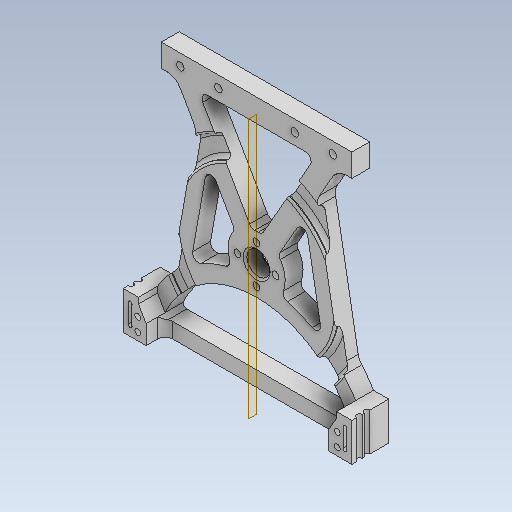
# Autodesk Inventor part: drv_stand_1
Saved by Autodesk Inventor 2020 (Build 240168000, 168)
## iProperties
Created: 2021-08-05
Part Number: drv_stand_1
Material: Generic
Document SubType Name: Modeling
Designer: Shuang Peng
Density: 1 g/cm^3
Appearance: Default
Author: Shuang Peng
Autodesk Inventor part; units mm, degrees
ref_plane "YZ Plane" through (0, 0, 0) normal (1, 0, 0) x (0, 1, 0)
ref_plane "XZ Plane" through (0, 0, 0) normal (0, 1, 0) x (-1, 0, 0)
ref_plane "XY Plane" through (0, 0, 0) normal (0, 0, 1) x (1, 0, 0)
sketch "Sketch1" plane through (0, 0, 0) normal (0, 0, 1) x (1, 0, 0)
  circle A0 centre (6, 23) radius 1.6 projected
  circle A1 centre (-6, 23) radius 1.6 projected
  arc A2 (-0.5, 30.4959) -> (0.5, 30.4959) centre (0, 0) ccw projected
  line L0 (0.5, 30.4959) -> (0.5, 11) projected
  arc A3 (-0.5, 11) -> (0.5, 11) centre (0, 11) ccw projected
  line L1 (-0.5, 11) -> (-0.5, 30.4959) projected
  circle A4 centre (-7, 0) radius 1.6 projected
  circle A5 centre (0, 7) radius 1.6 projected
  circle A6 centre (0, -7) radius 1.6 projected
  circle A7 centre (7, 0) radius 1.6 projected
  line L2 (-9.2147, 23.438) -> (-5.6564, 9.7982) projected
  arc A8 (-6.3264, 7.7445) -> (-5.6564, 9.7982) centre (-7.5917, 9.2933) ccw projected
  arc A9 (-6.3264, 7.7445) -> (-9.5652, 2.9167) centre (0, 0) ccw projected
  arc A10 (-11.4782, 1.5) -> (-9.5652, 2.9167) centre (-11.4782, 3.5) ccw projected
  line L3 (-11.4782, 1.5) -> (-25.2587, 1.5) projected
  arc A11 (-27.2397, 3.7745) -> (-25.2587, 1.5) centre (-25.2587, 3.5) ccw projected
  arc A12 (-12.0244, 24.7318) -> (-27.2397, 3.7745) centre (0, 0) ccw projected
  arc A13 (-9.2147, 23.438) -> (-12.0244, 24.7318) centre (-11.1499, 22.9332) ccw projected
  line L4 (-1.5, -11.4782) -> (-1.5, -25.2587) projected
  arc A14 (-3.7745, -27.2397) -> (-1.5, -25.2587) centre (-3.5, -25.2587) ccw projected
  arc A15 (-27.2397, -3.7745) -> (-3.7745, -27.2397) centre (0, 0) ccw projected
  arc A16 (-25.2587, -1.5) -> (-27.2397, -3.7745) centre (-25.2587, -3.5) ccw projected
  line L5 (-25.2587, -1.5) -> (-11.4782, -1.5) projected
  arc A17 (-9.5652, -2.9167) -> (-11.4782, -1.5) centre (-11.4782, -3.5) ccw projected
  arc A18 (-9.5652, -2.9167) -> (-2.9167, -9.5652) centre (0, 0) ccw projected
  arc A19 (-1.5, -11.4782) -> (-2.9167, -9.5652) centre (-3.5, -11.4782) ccw projected
  line L6 (5.6564, 9.7982) -> (9.2147, 23.438) projected
  arc A20 (12.0244, 24.7318) -> (9.2147, 23.438) centre (11.1499, 22.9332) ccw projected
  arc A21 (27.2397, 3.7745) -> (12.0244, 24.7318) centre (0, 0) ccw projected
  arc A22 (25.2587, 1.5) -> (27.2397, 3.7745) centre (25.2587, 3.5) ccw projected
  line L7 (25.2587, 1.5) -> (11.4782, 1.5) projected
  arc A23 (9.5652, 2.9167) -> (11.4782, 1.5) centre (11.4782, 3.5) ccw projected
  arc A24 (9.5652, 2.9167) -> (6.3264, 7.7445) centre (0, 0) ccw projected
  arc A25 (5.6564, 9.7982) -> (6.3264, 7.7445) centre (7.5917, 9.2933) ccw projected
  line L8 (1.5, -25.2587) -> (1.5, -11.4782) projected
  arc A26 (2.9167, -9.5652) -> (1.5, -11.4782) centre (3.5, -11.4782) ccw projected
  arc A27 (2.9167, -9.5652) -> (9.5652, -2.9167) centre (0, 0) ccw projected
  arc A28 (11.4782, -1.5) -> (9.5652, -2.9167) centre (11.4782, -3.5) ccw projected
  line L9 (11.4782, -1.5) -> (25.2587, -1.5) projected
  arc A29 (27.2397, -3.7745) -> (25.2587, -1.5) centre (25.2587, -3.5) ccw projected
  arc A30 (3.7745, -27.2397) -> (27.2397, -3.7745) centre (0, 0) ccw projected
  arc A31 (1.5, -25.2587) -> (3.7745, -27.2397) centre (3.5, -25.2587) ccw projected
  circle A32 centre (0, 0) radius 2 projected
  line L10 (0, 0) -> (-30, 0)
  line L11 (-30, 0) -> (-30, -20)
  line L12 (-30, -20) -> (-30, -28)
  line L13 (-30, -28) -> (-26, -28)
  line L14 (-26, -28) -> (-26, -18)
  line L15 (-26, -18) -> (-30, -18)
  line L16 (-30, -18) -> (-30, -28)
  dimension "d0" = 30
  dimension "d1" = 20
  dimension "d2" = 8
  dimension "d3" = 4
  dimension "d4" = 10
  constraints: 14 end point, 2 horizontal, 2 parallel, 2 vertical, 1 perpendicular
  measures "d0" distance of L10.start L10.end
  measures "d1" distance of L10.end L11.end
  measures "d2" distance of L11.end L12.end
  measures "d3" distance of L15.end L14.end
  measures "d4" distance of L14.end L13.end
ref_plane "Work Plane1" through (-30.5, -30.5, -4) normal (0, 0, -1) x (0, 1, 0)
extrude "Extrusion1" add sketch "Sketch1" against normal up to surface (4 mm away) contours L15 L14 L13 L12 L11
sketch "Sketch2" plane through (-26, -28, -4) normal (0, 0, -1) x (-1, 0, 0)
  line L0 (4, 0) -> (0, 0) projected
  line L1 (4, 10) -> (4, 0) projected
  line L2 (0, 10) -> (4, 10) projected
  line L3 (0, 0) -> (0, 10) projected
  line L4 (4, 0) -> (0, 0) projected
  line L5 (0, 0) -> (-2, 0)
  line L6 (-2, 0) -> (-2, 5)
  line L7 (-2, 5) -> (0, 8.4641)
  line L8 (0, 0) -> (0, 10) projected
  point P0 (-26, 28)
  point P1 (0, 8.4641)
  dimension "d7" = 2
  dimension "d8" = 5
  dimension "d9" = 30
  constraints: 6 end point, 1 horizontal, 1 parallel, 1 point on line
  measures "d7" distance of L0.end L5.end
  measures "d8" distance of L5.end L6.end
  measures "d9" angle of L3 L7
extrude "Extrusion2" add sketch "Sketch2" against normal up to surface (4 mm away) contours L5 L6 L7 L3
sketch "Sketch3" plane through (-26, -18, -4) normal (0, 0, -1) x (-1, 0, 0)
  line L0 (4, -10) -> (-2, -10) projected
  line L1 (4, 0) -> (4, -10) projected
  line L2 (0, 0) -> (4, 0) projected
  line L3 (0, -1.5359) -> (0, 0) projected
  line L4 (0, -1.5359) -> (-2, -5) projected
  line L5 (-2, -5) -> (-2, -10) projected
  line L6 (4, -10) -> (-2, -10) projected
  line L7 (-2, -10) -> (0.2, -10)
  line L8 (0.2, -10) -> (0.2, -8)
  line L9 (0.2, -8) -> (0.2, -4.5)
  circle A0 centre (0.2, -4.5) radius 0.75
  circle A1 centre (0.2, -8) radius 0.75
  point P0 (-26, 18)
  dimension "d12" = 2.2
  dimension "d13" = 2
  dimension "d14" = 3.5
  dimension "d15" = 1.5
  dimension "d16" = 1.5
  constraints: 6 end point, 2 centre point, 2 coincident, 2 point on line, 1 vertical
  measures "d12" distance of L0.end L7.end
  measures "d13" distance of L7.end L8.end
  measures "d14" distance of L8.end L9.end
  measures "d15" diameter of A0
  measures "d16" diameter of A1
extrude "Extrusion3" cut sketch "Sketch3" against normal blind 10 contours A1 L9 L8 | L8 L9 A1 | A0
ref_plane "Work Plane2" through (0, 30.996, -2) normal (-1, 0, 0) x (0, -1, 0)
mirror "Mirror1" about plane through (0, 30.996, -2) normal (-1, 0, 0) of "Extrusion1", "Extrusion2", "Extrusion3"
sketch "Sketch4" plane through (24, -28, -4) normal (0, 0, -1) x (-1, 0, 0)
  circle A0 centre (24, 28) radius 3.05
  circle A1 centre (24, 28) radius 7.5
  circle A2 centre (-2.2, 2) radius 0.75 projected
  circle A3 centre (-2.2, 5.5) radius 0.75 projected
  line L0 (-6, 0) -> (0, 0) projected
  line L1 (0, 5) -> (0, 0) projected
  line L2 (-2, 8.4641) -> (0, 5) projected
  line L3 (-2, 8.4641) -> (-2, 10) projected
  line L4 (-2, 10) -> (-6, 10) projected
  line L5 (-6, 10) -> (-6, 0) projected
  line L6 (54, 10) -> (54, 0) projected
  circle A4 centre (50.2, 2) radius 0.75 projected
  circle A5 centre (50.2, 5.5) radius 0.75 projected
  line L7 (54, 0) -> (48, 0) projected
  line L8 (54, 10) -> (54, 0) projected
  line L9 (50, 10) -> (54, 10) projected
  line L10 (50, 8.4641) -> (50, 10) projected
  line L11 (50, 8.4641) -> (48, 5) projected
  line L12 (48, 5) -> (48, 0) projected
  line L13 (0, 5) -> (0, 0) projected
  arc A6 (48, 5) -> (0, 5) centre (24, -5.8306) ccw
  line L14 (50, 10) -> (54, 10) projected
  line L15 (-2, 8.4641) -> (-2, 10) projected
  arc A7 (50, 10) -> (-2, 10) centre (24, -5.8306) ccw
  point P0 (30.3113, 23.9482)
  point P1 (17.6887, 23.9482)
  dimension "d19" = 6.1
  dimension "d20" = 15
  constraints: 4 centre point, 4 point on circle, 2 coincident, 1 concentric, 1 tangent
  measures "d19" diameter of A0
  measures "d20" diameter of A1
extrude "Extrusion4" add sketch "Sketch4" along normal blind 3
sketch "Sketch5" plane through (24, -28, -7) normal (0, 0, -1) x (-1, 0, 0)
  arc A0 (48, 5) -> (0, 5) centre (24, -5.8306) ccw projected
  line L0 (48, 5) -> (48, 0) projected
  line L1 (48, 0) -> (54, 0) projected
  line L2 (54, 0) -> (54, 10) projected
  line L3 (54, 10) -> (50, 10) projected
  arc A1 (50, 10) -> (30.3113, 23.9482) centre (24, -5.8306) ccw projected
  arc A2 (30.3113, 23.9482) -> (17.6887, 23.9482) centre (24, 28) ccw projected
  arc A3 (17.6887, 23.9482) -> (-2, 10) centre (24, -5.8306) ccw projected
  line L4 (-2, 10) -> (-6, 10) projected
  line L5 (-6, 10) -> (-6, 0) projected
  line L6 (-6, 0) -> (0, 0) projected
  line L7 (0, 0) -> (0, 5) projected
  circle A4 centre (24, 28) radius 3.05 projected
  circle A5 centre (50.2, 2) radius 0.75 projected
  circle A6 centre (50.2, 5.5) radius 0.75 projected
  circle A7 centre (-2.2, 5.5) radius 0.75 projected
  circle A8 centre (-2.2, 2) radius 0.75 projected
  circle A9 centre (24, 28) radius 5.55
  dimension "d23" = 2.5
  constraints: 1 centre point, 1 coincident
  measures "d23" radial gap between concentric circles of A4 A9
extrude "Extrusion5" add sketch "Sketch5" along normal blind 4 contours A9
sketch "Sketch6" plane through (24, -28, -7) normal (0, 0, -1) x (-1, 0, 0)
  circle A0 centre (24, 28) radius 5.55 projected
  arc A1 (48, 5) -> (0, 5) centre (24, -5.8306) ccw projected
  line L0 (48, 5) -> (48, 0) projected
  line L1 (48, 0) -> (54, 0) projected
  line L2 (54, 0) -> (54, 10) projected
  line L3 (54, 10) -> (50, 10) projected
  arc A2 (50, 10) -> (30.3113, 23.9482) centre (24, -5.8306) ccw projected
  arc A3 (30.3113, 23.9482) -> (17.6887, 23.9482) centre (24, 28) ccw projected
  arc A4 (17.6887, 23.9482) -> (-2, 10) centre (24, -5.8306) ccw projected
  line L4 (-2, 10) -> (-6, 10) projected
  line L5 (-6, 10) -> (-6, 0) projected
  line L6 (-6, 0) -> (0, 0) projected
  line L7 (0, 0) -> (0, 5) projected
  circle A5 centre (50.2, 2) radius 0.75 projected
  circle A6 centre (50.2, 5.5) radius 0.75 projected
  circle A7 centre (-2.2, 5.5) radius 0.75 projected
  circle A8 centre (-2.2, 2) radius 0.75 projected
  line L8 (-6, 0) -> (0, 0) projected
  line L9 (0, 0) -> (48, 0)
  line L10 (48, 0) -> (48, 4)
  line L11 (48, 4) -> (0, 4)
  line L12 (0, 4) -> (0, 0)
  point P0 (0, 4)
  dimension "d26" = 4
  constraints: 8 end point, 2 parallel, 1 horizontal, 1 perpendicular, 1 point on line
  measures "d26" distance between parallel lines of L9 L11
extrude "Extrusion6" add sketch "Sketch6" against normal blind 3 contours L0 L9 L7 L11
fillet "Fillet1" radius 1 2 edges at (-24, -24, -5.5) (24, -24, -5.5)
sketch "Sketch7" plane through (24, -28, -7) normal (0, 0, -1) x (-1, 0, 0)
  line L0 (24, 28) -> (24, 63)
  line L1 (-1, 60) -> (-1, 66)
  line L2 (-1, 66) -> (49, 66)
  line L3 (49, 66) -> (49, 60)
  line L4 (49, 60) -> (-1, 60)
  line L5 (-1, 60) -> (49, 66) construction
  line L6 (-1, 66) -> (49, 60) construction
  line L7 (-6, 0) -> (54, 0) projected
  line L8 (54, 0) -> (54, 10) projected
  line L9 (54, 10) -> (50, 10) projected
  arc A0 (50, 10) -> (30.3113, 23.9482) centre (24, -5.8306) ccw projected
  arc A1 (30.3113, 23.9482) -> (17.6887, 23.9482) centre (24, 28) ccw projected
  arc A2 (17.6887, 23.9482) -> (-2, 10) centre (24, -5.8306) ccw projected
  line L10 (-2, 10) -> (-6, 10) projected
  line L11 (-6, 10) -> (-6, 0) projected
  circle A3 centre (24, 28) radius 5.55 projected
  line L12 (47, 4) -> (1, 4) projected
  arc A4 (0, 5) -> (1, 4) centre (1, 5) ccw projected
  arc A5 (48, 5) -> (0, 5) centre (24, -5.8306) ccw projected
  arc A6 (47, 4) -> (48, 5) centre (47, 5) ccw projected
  circle A7 centre (50.2, 2) radius 0.75 projected
  circle A8 centre (50.2, 5.5) radius 0.75 projected
  circle A9 centre (-2.2, 5.5) radius 0.75 projected
  circle A10 centre (-2.2, 2) radius 0.75 projected
  line L13 (24, 63) -> (4, 63)
  line L14 (24, 28) -> (4, 63) construction
  line L15 (26.1706, 29.2403) -> (6.1706, 64.2403)
  line L16 (1.8294, 61.7597) -> (21.8294, 26.7597)
  arc A11 (21.8294, 26.7597) -> (26.1706, 29.2403) centre (24, 28) ccw
  arc A12 (6.1706, 64.2403) -> (1.8294, 61.7597) centre (4, 63) ccw
  line L17 (24, 63) -> (44, 63)
  circle A13 centre (24, 28) radius 5.55 projected
  line L18 (24, 28) -> (44, 63) construction
  line L19 (26.1706, 26.7597) -> (46.1706, 61.7597)
  line L20 (41.8294, 64.2403) -> (21.8294, 29.2403)
  arc A14 (21.8294, 29.2403) -> (26.1706, 26.7597) centre (24, 28) ccw
  arc A15 (46.1706, 61.7597) -> (41.8294, 64.2403) centre (44, 63) ccw
  point P0 (14, 45.5)
  point P1 (34, 45.5)
  point P2 (8.5937, 60)
  point P3 (39.4063, 60)
  point P4 (25.3376, 35.3798)
  point P5 (29.6788, 32.8991)
  point P6 (45.1651, 60)
  point P7 (2.8349, 60)
  point P8 (18.3212, 32.8991)
  point P9 (22.6624, 35.3798)
  dimension "d30" = 35
  dimension "d31" = 6
  dimension "d32" = 50
  dimension "d33" = 20
  dimension "d34" = 5
  dimension "d35" = 20
  dimension "d36" = 5
  constraints: 34 end point, 8 point on circle, 8 tangent, 5 parallel, 4 centre point, 4 midpoint, 2 perpendicular, 2 vertical
  measures "d30" distance of L0.start L0.end
  measures "d31" distance of L1.start L1.end
  measures "d32" distance of L1.end L2.end
  measures "d33" distance of L0.end L13.end
  measures "d34" diameter of A12
  measures "d35" distance of L0.end L17.end
  measures "d36" diameter of A15
extrude "Extrusion7" add sketch "Sketch7" against normal up to surface (3 mm away) contours A1 L16 L4 L15 | L20 L4 L19 A1 | L4 L15 L13 L0 | L0 L17 L20 L4 | L4 L16 A12 L15 | L20 A15 L19 L4 | L13 L15 A12 L16 L4 L1 L2 L3 L19 A15 L20 L17
sketch "Sketch8" plane through (24, -28, -4) normal (0, 0, 1) x (1, 0, 0)
  arc A0 (-22.6624, 35.3798) -> (-25.3376, 35.3798) centre (-24, 28) ccw projected
  line L0 (-25.3376, 35.3798) -> (-39.4063, 60) projected
  line L1 (-39.4063, 60) -> (-8.5937, 60) projected
  line L2 (-8.5937, 60) -> (-22.6624, 35.3798) projected
  line L3 (-18.3212, 32.8991) -> (-2.8349, 60) projected
  line L4 (-2.8349, 60) -> (1, 60) projected
  line L5 (1, 60) -> (1, 66) projected
  line L6 (1, 66) -> (-49, 66) projected
  line L7 (-49, 66) -> (-49, 60) projected
  line L8 (-49, 60) -> (-45.1651, 60) projected
  line L9 (-45.1651, 60) -> (-29.6788, 32.8991) projected
  arc A1 (-29.6788, 32.8991) -> (-30.3113, 23.9482) centre (-24, 28) ccw projected
  arc A2 (-30.3113, 23.9482) -> (-50, 10) centre (-24, -5.8306) ccw projected
  line L10 (-50, 8.4641) -> (-50, 10) projected
  line L11 (-50, 8.4641) -> (-48, 5) projected
  arc A3 (0, 5) -> (-48, 5) centre (-24, -5.8306) ccw projected
  line L12 (2, 8.4641) -> (0, 5) projected
  line L13 (2, 8.4641) -> (2, 10) projected
  arc A4 (2, 10) -> (-17.6887, 23.9482) centre (-24, -5.8306) ccw projected
  arc A5 (-17.6887, 23.9482) -> (-18.3212, 32.8991) centre (-24, 28) ccw projected
  circle A6 centre (-24, 28) radius 3.05 projected
  arc A7 (0, 5) -> (-48, 5) centre (-24, -5.8306) ccw projected
  line L14 (-2.9597, 10) -> (-11.1306, 55.5604) construction
  line L15 (-8.5937, 60) -> (-22.6624, 35.3798) projected
  line L16 (-0.9911, 10.3531) -> (-9.162, 55.9134)
  line L17 (-13.0992, 55.2073) -> (-4.9283, 9.6469)
  arc A8 (-4.9283, 9.6469) -> (-0.9911, 10.3531) centre (-2.9597, 10) ccw
  arc A9 (-9.162, 55.9134) -> (-13.0992, 55.2073) centre (-11.1306, 55.5604) ccw
  point P0 (-7.0452, 32.7802)
  point P1 (-11.3015, 45.1835)
  point P2 (-6.6365, 19.1717)
  point P3 (-1.8295, 15.0279)
  point P4 (-8.2084, 50.5963)
  dimension "d39" = 4
  constraints: 8 end point, 5 point on circle, 4 tangent, 2 centre point, 1 midpoint, 1 parallel, 1 point on line
  measures "d39" diameter of A9
extrude "Extrusion8" add sketch "Sketch8" against normal up to surface (3 mm away) contours L3 L16 A4 L17
mirror "Mirror2" about plane through (0, 30.996, -2) normal (-1, 0, 0) of "Extrusion8"
fillet "Fillet2" radius 1.5 12 edges at (17.3635, -8.8283, -5.5) (-17.3635, -8.8283, -5.5) (-12.6985, 17.1835, -5.5) (12.6985, 17.1835, -5.5) (6.3113, -4.0518, -5.5) (5.6788, 4.8991, -5.5) (-6.3113, -4.0518, -5.5) (-5.6788, 4.8991, -5.5) (-1.3376, 7.3798, -5.5) (1.3376, 7.3798, -5.5) (-15.4063, 32, -5.5) (15.4063, 32, -5.5)
fillet "Fillet3" radius 4 6 edges at (-22.1705, -12.9721, -5.5) (22.1705, -12.9721, -5.5) (15.7916, 22.5963, -5.5) (-15.7916, 22.5963, -5.5) (21.1651, 32, -5.5) (-21.1651, 32, -5.5)
sketch "Sketch9" plane through (-30, -28, 0) normal (0, -1, 0) x (1, 0, 0)
  line L0 (0, -1) -> (60, -1) projected
  line L1 (0, -3) -> (60, -3) projected
  line L2 (6, 0) -> (6, -4) projected
  line L3 (0, 0) -> (6, 0) projected
  line L4 (0, 0) -> (0, -7) projected
  line L5 (60, -7) -> (0, -7) projected
  line L6 (60, 0) -> (60, -7) projected
  line L7 (60, 0) -> (54, 0) projected
  line L8 (54, -4) -> (54, 0) projected
  line L9 (6, -4) -> (54, -4) projected
  circle A0 centre (0, -1) radius 0.75
  circle A1 centre (60, -3) radius 0.75
  point P0 (30, 0)
  dimension "d44" = 1.5
  dimension "d45" = 1.5
  constraints: 2 centre point, 2 coincident
  measures "d44" diameter of A0
  measures "d45" diameter of A1
extrude "Extrusion9" cut sketch "Sketch9" against normal up to surface (10 mm away) contours L4 A0 L0 | L4 A0 | L0 A0 L4 | A1 L6 | L6 L1 A1 | L1 L6 A1
fillet "Fillet4" radius 2 2 edges at (24, -25.5001, -4) (-24, -25.5, -4)
thicken "Thicken1" operation add thickness 4 both sides no extend neighbours yes toward (0, 0, 1) faces at (-4.6334, -0.686, -11)
sketch "Sketch10" plane through (25, 38, -7) normal (0, 0, -1) x (-1, 0, 0)
  line L0 (25, -38) -> (20, -38)
  circle A0 centre (20, -38) radius 0.9
  dimension "d54" = 5
  dimension "d55" = 1.8
  constraints: 2 end point, 1 centre point, 1 coincident, 1 horizontal
  measures "d54" distance of L0.start L0.end
  measures "d55" diameter of A0
extrude "Extrusion10" cut sketch "Sketch10" against normal blind 3
pattern_circular "Circular Pattern1" count 4 over 360 about axis through (0, 0, -4) along (0, 0, -1) of "Extrusion10"
mirror "Mirror3" about plane through (0, 30.996, -2) normal (-1, 0, 0) of "Extrusion9"
thicken "Thicken2" operation add thickness 1 both sides no extend neighbours yes toward (0, 0, 1) faces at (-28.9833, -22.8333, 0)
thicken "Thicken3" operation add thickness 1 both sides no extend neighbours yes toward (0, 0, 1) faces at (28.9833, -22.8333, 0)
sketch "Sketch12" plane through (24, -28, -4) normal (0, 0, 1) x (1, 0, 0)
  circle A0 centre (-24, 33) radius 0.9 projected
  circle A1 centre (-29, 28) radius 0.9 projected
  circle A2 centre (-24, 23) radius 0.9 projected
  circle A3 centre (-19, 28) radius 0.9 projected
  arc A4 (-46.8963, 14.2285) -> (-50, 10) centre (-24, -5.8306) ccw projected
  line L0 (-50, 8.4641) -> (-50, 10) projected
  line L1 (-50, 8.4641) -> (-48, 5) projected
  arc A5 (0, 5) -> (-48, 5) centre (-24, -5.8306) ccw projected
  line L2 (2, 8.4641) -> (0, 5) projected
  line L3 (2, 8.4641) -> (2, 10) projected
  arc A6 (2, 10) -> (-1.1037, 14.2285) centre (-24, -5.8306) ccw projected
  arc A7 (-2.0323, 16.1583) -> (-1.1037, 14.2285) centre (1.9049, 16.8644) ccw projected
  line L4 (-2.0323, 16.1583) -> (-7.952, 49.1667) projected
  arc A8 (-7.4878, 51.8574) -> (-7.952, 49.1667) centre (-4.0149, 49.8728) ccw projected
  line L5 (-7.4878, 51.8574) -> (-3.9866, 57.9846) projected
  arc A9 (-0.5136, 60) -> (-3.9866, 57.9846) centre (-0.5136, 56) ccw projected
  line L6 (-0.5136, 60) -> (1, 60) projected
  line L7 (1, 60) -> (1, 66) projected
  line L8 (1, 66) -> (-49, 66) projected
  line L9 (-49, 66) -> (-49, 60) projected
  line L10 (-49, 60) -> (-47.4864, 60) projected
  arc A10 (-44.0134, 57.9846) -> (-47.4864, 60) centre (-47.4864, 56) ccw projected
  line L11 (-44.0134, 57.9846) -> (-40.5122, 51.8574) projected
  arc A11 (-40.048, 49.1667) -> (-40.5122, 51.8574) centre (-43.9851, 49.8728) ccw projected
  line L12 (-45.9677, 16.1583) -> (-40.048, 49.1667) projected
  arc A12 (-46.8963, 14.2285) -> (-45.9677, 16.1583) centre (-49.9049, 16.8644) ccw projected
  arc A13 (-17.8294, 33.7597) -> (-17.7725, 32.1795) centre (-16.527, 33.0154) ccw projected
  line L13 (-17.8294, 33.7597) -> (-13.3511, 41.5967) projected
  arc A14 (-10.5723, 41.1173) -> (-13.3511, 41.5967) centre (-12.0487, 40.8525) ccw projected
  line L14 (-10.5723, 41.1173) -> (-7.2288, 22.4743) projected
  arc A15 (-9.4235, 20.8927) -> (-7.2288, 22.4743) centre (-8.7052, 22.2095) ccw projected
  arc A16 (-9.4235, 20.8927) -> (-15.925, 23.519) centre (-24, -5.8306) ccw projected
  arc A17 (-16.9392, 25.4711) -> (-15.925, 23.519) centre (-15.5271, 24.9653) ccw projected
  arc A18 (-16.9392, 25.4711) -> (-17.7725, 32.1795) centre (-24, 28) ccw projected
  line L15 (-34.6489, 41.5967) -> (-30.1706, 33.7597) projected
  arc A19 (-30.2275, 32.1795) -> (-30.1706, 33.7597) centre (-31.473, 33.0154) ccw projected
  arc A20 (-30.2275, 32.1795) -> (-31.0608, 25.4711) centre (-24, 28) ccw projected
  arc A21 (-32.075, 23.519) -> (-31.0608, 25.4711) centre (-32.4729, 24.9653) ccw projected
  arc A22 (-32.075, 23.519) -> (-38.5765, 20.8927) centre (-24, -5.8306) ccw projected
  arc A23 (-40.7712, 22.4743) -> (-38.5765, 20.8927) centre (-39.2948, 22.2095) ccw projected
  line L16 (-37.4277, 41.1173) -> (-40.7712, 22.4743) projected
  arc A24 (-34.6489, 41.5967) -> (-37.4277, 41.1173) centre (-35.9513, 40.8525) ccw projected
  line L17 (-25.8294, 36.2403) -> (-38.1239, 57.7558) projected
  arc A25 (-36.8216, 60) -> (-38.1239, 57.7558) centre (-36.8216, 58.5) ccw projected
  line L18 (-36.8216, 60) -> (-11.1784, 60) projected
  arc A26 (-9.8761, 57.7558) -> (-11.1784, 60) centre (-11.1784, 58.5) ccw projected
  line L19 (-9.8761, 57.7558) -> (-22.1706, 36.2403) projected
  arc A27 (-23.5608, 35.4871) -> (-22.1706, 36.2403) centre (-23.473, 36.9846) ccw projected
  arc A28 (-23.5608, 35.4871) -> (-24.4392, 35.4871) centre (-24, 28) ccw projected
  arc A29 (-25.8294, 36.2403) -> (-24.4392, 35.4871) centre (-24.527, 36.9846) ccw projected
  circle A30 centre (-24, 28) radius 3.05 projected
  line L20 (-49, 60) -> (-49, 66) projected
  line L21 (-49, 63) -> (-44, 63)
  circle A31 centre (-44, 63) radius 1
  line L22 (1, 60) -> (1, 66) projected
  line L23 (1, 63) -> (-4, 63)
  circle A32 centre (-4, 63) radius 1
  line L24 (-44, 63) -> (-34, 63)
  circle A33 centre (-34, 63) radius 1
  line L25 (-4, 63) -> (-14, 63)
  circle A34 centre (-14, 63) radius 1
  dimension "d74" = 5
  dimension "d75" = 2
  dimension "d76" = 5
  dimension "d77" = 2
  dimension "d78" = 10
  dimension "d79" = 2
  dimension "d80" = 10
  dimension "d81" = 2
  constraints: 8 end point, 4 centre point, 4 coincident, 3 horizontal, 2 midpoint, 1 point on line
  measures "d74" distance of L21.start L21.end
  measures "d75" diameter of A31
  measures "d76" distance of L23.start L23.end
  measures "d77" diameter of A32
  measures "d78" distance of L24.start L24.end
  measures "d79" diameter of A33
  measures "d80" distance of L25.start L25.end
  measures "d81" diameter of A34
extrude "Extrusion12" cut sketch "Sketch12" against normal blind 9 contours A31 L24 L21 | L21 L24 A31 | A32 L25 L23 | L23 L25 A32 | A33 | A34
sketch "Sketch13" plane through (24, -28, -4) normal (0, 0, 1) x (1, 0, 0)
  circle A0 centre (-14, 63) radius 1 projected
  circle A1 centre (-34, 63) radius 1 projected
  circle A2 centre (-4, 63) radius 1 projected
  circle A3 centre (-44, 63) radius 1 projected
  circle A4 centre (-24, 33) radius 0.9 projected
  circle A5 centre (-29, 28) radius 0.9 projected
  circle A6 centre (-24, 23) radius 0.9 projected
  circle A7 centre (-19, 28) radius 0.9 projected
  arc A8 (-46.8963, 14.2285) -> (-50, 10) centre (-24, -5.8306) ccw projected
  line L0 (-50, 8.4641) -> (-50, 10) projected
  line L1 (-50, 8.4641) -> (-48, 5) projected
  arc A9 (0, 5) -> (-48, 5) centre (-24, -5.8306) ccw projected
  line L2 (2, 8.4641) -> (0, 5) projected
  line L3 (2, 8.4641) -> (2, 10) projected
  arc A10 (2, 10) -> (-1.1037, 14.2285) centre (-24, -5.8306) ccw projected
  arc A11 (-2.0323, 16.1583) -> (-1.1037, 14.2285) centre (1.9049, 16.8644) ccw projected
  line L4 (-2.0323, 16.1583) -> (-7.952, 49.1667) projected
  arc A12 (-7.4878, 51.8574) -> (-7.952, 49.1667) centre (-4.0149, 49.8728) ccw projected
  line L5 (-7.4878, 51.8574) -> (-3.9866, 57.9846) projected
  arc A13 (-0.5136, 60) -> (-3.9866, 57.9846) centre (-0.5136, 56) ccw projected
  line L6 (-0.5136, 60) -> (1, 60) projected
  line L7 (1, 60) -> (1, 66) projected
  line L8 (1, 66) -> (-49, 66) projected
  line L9 (-49, 66) -> (-49, 60) projected
  line L10 (-49, 60) -> (-47.4864, 60) projected
  arc A14 (-44.0134, 57.9846) -> (-47.4864, 60) centre (-47.4864, 56) ccw projected
  line L11 (-44.0134, 57.9846) -> (-40.5122, 51.8574) projected
  arc A15 (-40.048, 49.1667) -> (-40.5122, 51.8574) centre (-43.9851, 49.8728) ccw projected
  line L12 (-45.9677, 16.1583) -> (-40.048, 49.1667) projected
  arc A16 (-46.8963, 14.2285) -> (-45.9677, 16.1583) centre (-49.9049, 16.8644) ccw projected
  arc A17 (-17.8294, 33.7597) -> (-17.7725, 32.1795) centre (-16.527, 33.0154) ccw projected
  line L13 (-17.8294, 33.7597) -> (-13.3511, 41.5967) projected
  arc A18 (-10.5723, 41.1173) -> (-13.3511, 41.5967) centre (-12.0487, 40.8525) ccw projected
  line L14 (-10.5723, 41.1173) -> (-7.2288, 22.4743) projected
  arc A19 (-9.4235, 20.8927) -> (-7.2288, 22.4743) centre (-8.7052, 22.2095) ccw projected
  arc A20 (-9.4235, 20.8927) -> (-15.925, 23.519) centre (-24, -5.8306) ccw projected
  arc A21 (-16.9392, 25.4711) -> (-15.925, 23.519) centre (-15.5271, 24.9653) ccw projected
  arc A22 (-16.9392, 25.4711) -> (-17.7725, 32.1795) centre (-24, 28) ccw projected
  line L15 (-34.6489, 41.5967) -> (-30.1706, 33.7597) projected
  arc A23 (-30.2275, 32.1795) -> (-30.1706, 33.7597) centre (-31.473, 33.0154) ccw projected
  arc A24 (-30.2275, 32.1795) -> (-31.0608, 25.4711) centre (-24, 28) ccw projected
  arc A25 (-32.075, 23.519) -> (-31.0608, 25.4711) centre (-32.4729, 24.9653) ccw projected
  arc A26 (-32.075, 23.519) -> (-38.5765, 20.8927) centre (-24, -5.8306) ccw projected
  arc A27 (-40.7712, 22.4743) -> (-38.5765, 20.8927) centre (-39.2948, 22.2095) ccw projected
  line L16 (-37.4277, 41.1173) -> (-40.7712, 22.4743) projected
  arc A28 (-34.6489, 41.5967) -> (-37.4277, 41.1173) centre (-35.9513, 40.8525) ccw projected
  line L17 (-25.8294, 36.2403) -> (-38.1239, 57.7558) projected
  arc A29 (-36.8216, 60) -> (-38.1239, 57.7558) centre (-36.8216, 58.5) ccw projected
  line L18 (-36.8216, 60) -> (-11.1784, 60) projected
  arc A30 (-9.8761, 57.7558) -> (-11.1784, 60) centre (-11.1784, 58.5) ccw projected
  line L19 (-9.8761, 57.7558) -> (-22.1706, 36.2403) projected
  arc A31 (-23.5608, 35.4871) -> (-22.1706, 36.2403) centre (-23.473, 36.9846) ccw projected
  arc A32 (-23.5608, 35.4871) -> (-24.4392, 35.4871) centre (-24, 28) ccw projected
  arc A33 (-25.8294, 36.2403) -> (-24.4392, 35.4871) centre (-24.527, 36.9846) ccw projected
  circle A34 centre (-24, 28) radius 3.05 projected
  circle A35 centre (-18, 51) radius 1.6 projected
  circle A36 centre (-24, 28) radius 3.05 projected
  circle A37 centre (-24, 28) radius 21
  circle A38 centre (-24, 28) radius 26.5
  point P0 (-34.9184, 52.1462)
  point P1 (-40.0643, 49.0758)
  point P2 (-41.8642, 39.0395)
  point P3 (-32.1742, 47.3438)
  point P4 (-46.7485, 14.4074)
  point P5 (-44.2887, 10.9524)
  point P6 (-40.3438, 14.8136)
  point P7 (-44.5872, 23.8564)
  point P8 (-3.7113, 10.9524)
  point P9 (-1.2515, 14.4074)
  point P10 (-3.4128, 23.8564)
  point P11 (-7.6562, 14.8136)
  point P12 (-7.9357, 49.0758)
  point P13 (-13.0816, 52.1462)
  point P14 (-15.8258, 47.3438)
  point P15 (-6.1358, 39.0395)
  dimension "d84" = 42
  dimension "d85" = 53
  constraints: 2 centre point, 2 coincident
  measures "d84" diameter of A37
  measures "d85" diameter of A38
extrude "Extrusion13" cut sketch "Sketch13" against normal blind 1.7 contours A16 L12 A37 A9 A38 | A38 L17 A37 L12 | A9 A37 L4 A11 A38 | A38 L4 A37 L19
fillet "Fillet5" radius 1 8 edges at (-13.6653, 15.9455, -5.7) (-13.5784, 22.7569, -5.7) (13.5784, 22.7569, -5.7) (13.6653, 15.9455, -5.7) (19.011, -8.921, -5.7) (21.5878, -15.3693, -5.7) (-21.5878, -15.3693, -5.7) (-19.011, -8.921, -5.7)
fillet "Fillet6" radius 0.5 8 edges at (13.5784, 22.7569, -4) (13.6653, 15.9455, -4) (19.011, -8.921, -4) (21.5878, -15.3693, -4) (-21.5878, -15.3693, -4) (-19.011, -8.921, -4) (-13.6653, 15.9455, -4) (-13.5784, 22.7569, -4)
thicken "Thicken4" operation add thickness 1.7 both sides no extend neighbours yes toward (0, 0, -1) faces at (-17.1478, 7.4808, -7)
chamfer "Chamfer4" distance 0.5 angle 45 2 edges at (3.05, 0, -8.7) (3.05, 0, -4)
sketch "Sketch14" plane through (-30, -18, 1) normal (0, 0, 1) x (1, 0, 0)
  circle A0 centre (3.8, -8) radius 0.75 projected
  circle A1 centre (3.8, -4.5) radius 0.75 projected
  line L0 (0, 0) -> (0, -10) projected
  line L1 (0, -10) -> (6, -10) projected
  line L2 (6, -5) -> (6, -10) projected
  line L3 (4, -1.5359) -> (6, -5) projected
  line L4 (4, -1.5359) -> (4, 0) projected
  line L5 (4, 0) -> (0, 0) projected
  line L6 (0.75, -10) -> (0.75, 0) projected
  line L7 (3.8, -8) -> (3.8, -4.5)
  line L8 (3.8, -4.5) -> (3.8, -5)
  line L9 (3.8, -5) -> (1.8, -5)
  line L10 (1.8, -2.5) -> (1.8, -7.5) construction
  line L11 (1.3, -2.5) -> (1.3, -7.5)
  line L12 (2.3, -7.5) -> (2.3, -2.5)
  arc A2 (2.3, -2.5) -> (1.3, -2.5) centre (1.8, -2.5) ccw
  arc A3 (1.3, -7.5) -> (2.3, -7.5) centre (1.8, -7.5) ccw
  point P0 (30, 18)
  dimension "d98" = 0.5
  dimension "d99" = 2
  dimension "d100" = 2.5
  dimension "d101" = 1
  constraints: 14 end point, 4 point on circle, 4 tangent, 2 centre point, 2 vertical, 1 midpoint, 1 parallel, 1 perpendicular, 1 point on line
  measures "d98" distance of L7.end L8.end
  measures "d99" distance of L8.end L9.end
  measures "d100" distance of L9.end L10.end
  measures "d101" diameter of A3
extrude "Extrusion14" cut sketch "Sketch14" against normal blind 20 contours A2 L12 A3 L11
mirror "Mirror5" about plane through (0, 30.996, -2) normal (-1, 0, 0) of "Extrusion14"
body "Solid1"
